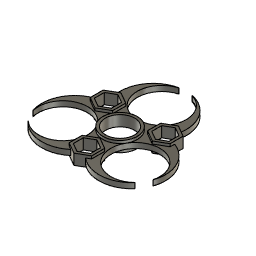
fidget spinner (Autodesk Fusion 360 design; units mm, degrees)
Autodesk Fusion 360 part; units mm, degrees
sketch "Sketch1" plane through (0, 0, 0) normal (0, 0, 1) x (1, 0, 0)
  circle A0 centre (0, 0) radius 50 construction
  line L0 (0, 103.6273) -> (0, -40.6273) construction
  circle A1 centre (0, 0) radius 11
  circle A2 centre (0, 0) radius 13
  circle A3 centre (0, 25) radius 25
  line L1 (-60, 0) -> (67.6208, 0) construction
  circle A4 centre (0, 31.5) radius 18.5
  line L2 (-5, 70) -> (5, 70)
  line L3 (5, 70) -> (5, 0)
  line L4 (5, 0) -> (-5, 0)
  line L5 (-5, 0) -> (-5, 70)
  circle A5 centre (-27.2798, -15.75) radius 18.5
  circle A6 centre (-21.6506, -12.5) radius 25
  line L6 (2.5, -4.3301) -> (-58.1218, -39.3301)
  line L7 (-63.1218, -30.6699) -> (-2.5, 4.3301)
  line L8 (-58.1218, -39.3301) -> (-63.1218, -30.6699)
  circle A7 centre (27.2798, -15.75) radius 18.5
  circle A8 centre (21.6506, -12.5) radius 25
  line L9 (2.5, 4.3301) -> (63.1218, -30.6699)
  line L10 (58.1218, -39.3301) -> (-2.5, -4.3301)
  line L11 (63.1218, -30.6699) -> (58.1218, -39.3301)
  point P0 (0, 50)
  dimension "d2" = 100
  dimension "d3" = 22
  dimension "d4" = 2
  dimension "d8" = 10
  dimension "d9" = 70
  dimension "d11" = 360
  constraint coincident A0.centre A1.centre
  constraint vertical L0
  constraint coincident L0 A3.centre
  constraint tangent A0 A3
  constraint horizontal L1
  constraint coincident A0.centre L1
  constraint coincident L0 A0.centre
  constraint tangent A3 L1
  constraint tangent A2 A4
  constraint tangent A3 A4
  constraint midpoint L0 A4.centre
  constraint coincident L0 P0
  constraint coincident A3 P0
  constraint horizontal L2
  constraint vertical L3
  constraint horizontal L4
  constraint vertical L5
  constraint coincident L1 L3.end
  constraint midpoint A0.centre L4
  measures "d2" diameter of A0
  measures "d3" diameter of A1
  measures "d8" distance of L2.start L2.end
  measures "d9" distance of L2.start L4.end
extrude "Extrude1" add sketch "Sketch1" along normal mid plane 8 contours A1 A2 A3 L9 | A1 A2 A3 A8 | A1 A2 L9 L10 | A1 A2 L3 A8 | A1 A2 A6 L10 | A1 A2 L3 L5 | A1 A2 A6 A8 | A1 A2 L5 A6 | A1 A2 L6 A8 | A1 A2 A3 A6 | A1 A2 L6 L7 | A1 A2 A3 L7
extrude "Extrude2" add sketch "Sketch1" along normal mid plane 4 contours A2 A3 A7 A8 L9 | A2 A3 A8 | A2 A7 L9 | A2 A3 A4 L3 A8 | A2 A6 A7 A8 L10 | A2 A7 L10 | A2 A4 L3 | A2 A6 A8 | A2 A4 L5 | A2 A3 A4 L5 A6 | A2 A5 A6 L6 A8 | A2 A3 A6 | A2 A5 L6 | A2 A3 A5 A6 L7 | A2 A5 L7
sketch "Sketch2" plane through (0, 0, 2) normal (0, 0, 1) x (-1, 0, 0)
  line L0 (-45.205, 20.3256) -> (-45.3638, 20.4173)
  arc A0 (-45.3638, 20.4173) -> (-21.6506, -12.5) centre (-21.6506, 12.5) ccw
  arc A1 (-21.6506, -12.5) -> (-5, -49.4949) centre (0, -25) ccw
  line L1 (-5, -49.4949) -> (-5, -49.3115)
  arc A2 (0, -13) -> (-5, -49.3115) centre (0, -31.5) ccw
  arc A3 (-11.2583, 6.5) -> (0, -13) centre (0, 0) ccw
  arc A4 (-45.205, 20.3256) -> (-11.2583, 6.5) centre (-27.2798, 15.75) ccw
  line L2 (0, 0) -> (-21.6506, -12.5) construction
  line L3 (-40.2014, -23.2103) -> (-21.6506, -12.5) construction
  line L4 (-28.1506, -8.7472) -> (-28.1506, -16.2528)
  line L5 (-28.1506, -16.2528) -> (-21.6506, -20.0056)
  line L6 (-21.6506, -20.0056) -> (-15.1506, -16.2528)
  line L7 (-15.1506, -16.2528) -> (-15.1506, -8.7472)
  line L8 (-15.1506, -8.7472) -> (-21.6506, -4.9944)
  line L9 (-21.6506, -4.9944) -> (-28.1506, -8.7472)
  line L10 (-13.1506, -7.5925) -> (-21.6506, -2.685)
  line L11 (-21.6506, -2.685) -> (-30.1506, -7.5925)
  line L12 (-30.1506, -7.5925) -> (-30.1506, -17.4075)
  line L13 (-30.1506, -17.4075) -> (-21.6506, -22.315)
  line L14 (-21.6506, -22.315) -> (-13.1506, -17.4075)
  line L15 (-13.1506, -17.4075) -> (-13.1506, -7.5925)
  line L16 (30.1506, -7.5925) -> (21.6506, -2.685)
  line L17 (13.1506, -17.4075) -> (21.6506, -22.315)
  line L18 (15.1506, -8.7472) -> (15.1506, -16.2528)
  line L19 (15.1506, -16.2528) -> (21.6506, -20.0056)
  line L20 (13.1506, -7.5925) -> (13.1506, -17.4075)
  line L21 (21.6506, -22.315) -> (30.1506, -17.4075)
  line L22 (21.6506, -20.0056) -> (28.1506, -16.2528)
  line L23 (28.1506, -16.2528) -> (28.1506, -8.7472)
  line L24 (30.1506, -17.4075) -> (30.1506, -7.5925)
  line L25 (28.1506, -8.7472) -> (21.6506, -4.9944)
  line L26 (21.6506, -2.685) -> (13.1506, -7.5925)
  line L27 (21.6506, -4.9944) -> (15.1506, -8.7472)
  line L28 (-8.5, 29.9075) -> (-8.5, 20.0925)
  line L29 (8.5, 20.0925) -> (8.5, 29.9075)
  line L30 (0, 17.4944) -> (6.5, 21.2472)
  line L31 (6.5, 21.2472) -> (6.5, 28.7528)
  line L32 (0, 15.185) -> (8.5, 20.0925)
  line L33 (8.5, 29.9075) -> (0, 34.815)
  line L34 (6.5, 28.7528) -> (0, 32.5056)
  line L35 (0, 32.5056) -> (-6.5, 28.7528)
  line L36 (0, 34.815) -> (-8.5, 29.9075)
  line L37 (-6.5, 28.7528) -> (-6.5, 21.2472)
  line L38 (-8.5, 20.0925) -> (0, 15.185)
  line L39 (-6.5, 21.2472) -> (0, 17.4944)
  point P0 (-21.6506, -12.5)
  point P1 (21.6506, -12.5)
  point P2 (21.6506, -12.5)
  point P3 (21.6506, -12.5)
  point P4 (0, 25)
  point P5 (0, 25)
  point P6 (0, 25)
  dimension "d16" = 6.5
  dimension "d17" = 2
  dimension "d19" = 360
  constraint coincident A3.centre L2.start
  constraint coincident P0 A0.end
  constraint parallel L2 L3
  constraint coincident L3 L4.end
  measures "d16" distance of P0 L9
extrude "Extrude3" add sketch "Sketch2" along normal blind 2 and the other way blind 6 contours A0 A1 L4 L5 L6 L7 L8 L9 L10 L11 L12 L13 L14 L15 | A0 A1 L4 L5 L12 L13 | L16 L17 L20 L21 L24 L26 | L28 L29 L32 L33 L36 L38
extrude "Extrude4" cut 3 faces at (-17.3173, 12.5, 2) (-2.1667, -21.2472, 2) (19.484, 8.7472, 2) along direction (0, 0, -1) blind 20
